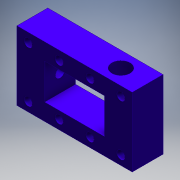
# Autodesk Inventor part: Distributore
Saved by Autodesk Inventor 2016 (Build 200138000, 138)
## iProperties
Created: 2016-09-10
Part Number: Distributore
Material: Generic
Document SubType Name: Modeling
Designer: Muhammad
Density: 1 g/cm^3
Appearance: Default
Author: Muhammad
Autodesk Inventor part; units mm, degrees
ref_plane "YZ Plane" through (0, 0, 0) normal (1, 0, 0) x (0, 1, 0)
ref_plane "XZ Plane" through (0, 0, 0) normal (0, 1, 0) x (-1, 0, 0)
ref_plane "XY Plane" through (0, 0, 0) normal (0, 0, 1) x (1, 0, 0)
sketch "Sketch1" plane through (0, 0, 0) normal (0, 1, 0) x (-1, 0, 0)
  line L0 (31.75, 19) -> (-31.75, 19)
  line L1 (-31.75, 19) -> (-31.75, -19)
  line L2 (-31.75, -19) -> (31.75, -19)
  line L3 (31.75, -19) -> (31.75, 19)
  line L4 (31.75, 19) -> (31.75, 14) construction
  line L5 (31.75, 14) -> (31.75, -14) construction
  line L6 (31.75, 19) -> (25.5, 19) construction
  line L7 (25.5, 19) -> (8.5, 19) construction
  line L8 (8.5, 19) -> (-8.5, 19) construction
  line L9 (-8.5, 19) -> (-25.5, 19) construction
  line L10 (31.75, 14) -> (-25.5, 14) construction
  line L11 (-25.5, 14) -> (-25.5, -14) construction
  line L12 (-25.5, -14) -> (-8.5, -14) construction
  line L13 (-8.5, -14) -> (8.5, -14) construction
  line L14 (8.5, -14) -> (25.5, -14) construction
  line L15 (25.5, -14) -> (31.75, -14) construction
  line L16 (25.5, 14) -> (25.5, -14) construction
  line L17 (8.5, 14) -> (8.5, -14) construction
  line L18 (-8.5, 14) -> (-8.5, -14) construction
  circle A0 centre (25.5, 14) radius 2.25
  circle A1 centre (25.5, -14) radius 2.25
  circle A2 centre (8.5, -14) radius 2.25
  circle A3 centre (-8.5, -14) radius 2.25
  circle A4 centre (-25.5, -14) radius 2.25
  circle A5 centre (-25.5, 14) radius 2.25
  circle A6 centre (-8.5, 14) radius 2.25
  circle A7 centre (8.5, 14) radius 2.25
  point P0 (0, 0)
  dimension "d0" = 63.5
  dimension "d1" = 38
  dimension "d5" = 17
  dimension "d6" = 17
  dimension "d7" = 17
  constraints: 38 end point, 11 point on line, 8 centre point, 8 coincident, 6 perpendicular, 3 parallel, 1 collinear, 1 horizontal
  measures "d0" distance of L2.end L1.end
  measures "d1" distance of L1.end L0.end
  measures "d5" distance of L6.end L7.end
  measures "d6" distance of L7.end L8.end
  measures "d7" distance of L8.end L9.end
extrude "Extrusion1" add sketch "Sketch1" along normal blind 17
sketch "Sketch2" plane through (0, 17, 0) normal (0, 1, 0) x (1, 0, 0)
  line L0 (-16.5, -9.75) -> (16.5, -9.75)
  line L1 (16.5, -9.75) -> (16.5, 9.75)
  line L2 (16.5, 9.75) -> (-16.5, 9.75)
  line L3 (-16.5, 9.75) -> (-16.5, -9.75)
  line L4 (-16.5, -9.75) -> (16.5, 9.75) construction
  line L5 (16.5, -9.75) -> (-16.5, 9.75) construction
  point P0 (0, 0)
  dimension "d12" = 33
  dimension "d13" = 19.5
  constraints: 12 end point, 2 midpoint, 2 parallel, 1 horizontal, 1 perpendicular
  measures "d12" distance of L2.end L1.end
  measures "d13" distance of L1.end L0.end
extrude "Extrusion2" cut sketch "Sketch2" against normal through all
sketch "Sketch3" plane through (-31.75, 0, -19) normal (-1, 0, 0) x (0, 0, 1)
  line L0 (19, 0) -> (19, 17) construction
  line L1 (38, 17) -> (0, 17) construction
  line L2 (0, 0) -> (0, 17) construction
  line L3 (0, 8.5) -> (38, 8.5) construction
  line L4 (38, 0) -> (38, 17) construction
  circle A0 centre (19, 8.5) radius 2.08 construction
  constraints: 4 end point, 4 midpoint, 1 centre point
hole "Hole1" at (-31.75, 8.5, 0) direction (1, 0, 0) diameter 10 depth 8.6 tip angle 118
sketch "Sketch4" plane through (-16.5, 17, 9.75) normal (1, 0, 0) x (0, 0, -1)
  line L0 (-9.25, -17) -> (-9.25, 0) construction
  line L1 (-9.25, -8.5) -> (28.75, -8.5) construction
  line L2 (28.75, -17) -> (28.75, 0) construction
  circle A0 centre (9.75, -8.5) radius 2.55
  point P0 (9.75, -17)
  dimension "d23" = 5.1
  constraints: 3 midpoint, 2 end point, 1 centre point
  measures "d23" diameter of A0
extrude "Extrusion3" cut sketch "Sketch4" against normal through all
sketch "Sketch5" plane through (-31.75, 0, 19) normal (0, 0, 1) x (1, 0, 0)
  line L0 (63.5, 0) -> (63.5, 17) construction
  line L1 (63.5, 8.5) -> (48.8, 8.5) construction
  circle A0 centre (48.8, 8.5) radius 5
  point P0 (31.75, 0)
  dimension "d26" = 14.7
  dimension "d27" = 10
  constraints: 2 end point, 1 centre point, 1 coincident, 1 horizontal, 1 midpoint
  measures "d26" distance of L1.start L1.end
  measures "d27" diameter of A0
extrude "Extrusion4" cut sketch "Sketch5" against normal blind 10
sketch "Sketch6" plane through (-31.75, 0, 19) normal (0, 0, 1) x (1, 0, 0)
  line L0 (63.5, 0) -> (63.5, 17) construction
  line L1 (63.5, 8.5) -> (48.8, 8.5) construction
  point P0 (31.75, 0)
  dimension "d30" = 14.7
  constraints: 2 end point, 1 horizontal, 1 midpoint
  measures "d30" distance of L1.start L1.end
hole "Hole2" at (17.05, 8.5, 19) direction (0, 0, -1) diameter 9.5 depth 17 tip angle 118
body "Solid1"
